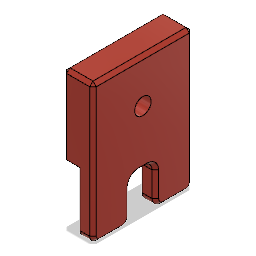
Bearing-mounting-blockV2 v6 (Autodesk Fusion 360 design; units mm, degrees)
Autodesk Fusion 360 part; units mm, degrees
sketch "Sketch1" plane through (0, 0, 0) normal (1, 0, 0) x (0, 0, -1)
  circle A0 centre (0, 0) radius 5
  line L0 (-30.15, -21.15) -> (30.15, -21.15)
  line L1 (30.15, -21.15) -> (30.15, 21.15)
  line L2 (-30.15, -21.15) -> (-30.15, 26.15)
  line L3 (-30.15, 26.15) -> (30.15, 26.15)
  line L4 (30.15, 26.15) -> (30.15, 21.15)
  dimension "d11" = 10
  dimension "d127" = 60.3
  dimension "d142" = 21.15
  dimension "d143" = 30.15
  measures "d11" diameter of A0
  measures "d127" distance of L2 L4
extrude "Extrude1" add sketch "Sketch1" along normal blind 8
sketch "Sketch16" plane through (0, -21.15, 0) normal (0, -1, 0) x (1, 0, 0)
  line L0 (0, 30.15) -> (0, -30.15)
  line L1 (0, -30.15) -> (8, -30.15)
  line L2 (8, -30.15) -> (8, 30.15)
  line L3 (8, 30.15) -> (0, 30.15)
  line L4 (4, 26.25) -> (4, -26.25) construction
  circle A0 centre (4, 26.25) radius 2.6
  circle A1 centre (4, -26.25) radius 2.6
  dimension "d144" = 4
  dimension "d145" = 52.5
  dimension "d146" = 5.2
  dimension "d147" = 5.2
  dimension "d148" = 26.25
  measures "d144" distance of origin L4
  measures "d146" diameter of A0
  measures "d147" diameter of A1
  measures "d148" distance of origin
extrude "Extrude17" cut sketch "Sketch16" against normal blind 7 contours A0 | A1
sketch "Sketch17" plane through (0, -14.15, 0) normal (0, -1, 0) x (1, 0, 0)
  circle A0 centre (4, 26.25) radius 2.6
  line L0 (4, 26.25) -> (4, -26.25)
  circle A1 centre (4, 26.25) radius 2
  circle A2 centre (4, -26.25) radius 2
  dimension "d151" = 52.5
  dimension "d152" = 4
  dimension "d153" = 4
  measures "d152" diameter of A2
  measures "d153" diameter of A1
extrude "Extrude18" cut sketch "Sketch17" against normal blind 10 contours A1 | A2
extrude "Extrude19" add 1 faces at (8, 1.9151, -21.7481) along direction (1, 0, 0) blind 10
sketch "Sketch18" plane through (0, -21.15, 0) normal (0, -1, 0) x (1, 0, 0)
  circle A0 centre (4, 26.25) radius 2.6
  circle A1 centre (4, -26.25) radius 2.6
  line L0 (0, 30.15) -> (0, -30.15)
  line L1 (0, -30.15) -> (18, -30.15)
  line L2 (18, -30.15) -> (18, 30.15)
  line L3 (18, 30.15) -> (0, 30.15)
  line L4 (18, 30.15) -> (8, 30.15)
  line L5 (8, 30.15) -> (8, -30.15)
  line L6 (8, -30.15) -> (18, -30.15)
  line L7 (18, -30.15) -> (18, 30.15)
  dimension "d159" = 10
  measures "d159" distance of L5 L7
extrude "Extrude20" add sketch "Sketch18" along normal blind 37 contours L1 L2 L3 L4 L5 L6 L7
sketch "Sketch19" plane through (18, 0, 0) normal (1, 0, 0) x (0, 0, -1)
  circle A0 centre (0, 0) radius 5
  line L0 (30.15, -58.15) -> (30.15, 26.15)
  line L1 (30.15, 26.15) -> (-30.15, 26.15)
  line L2 (-30.15, 26.15) -> (-30.15, -58.15)
  line L3 (-7.5, -58.15) -> (7.5, -58.15)
  line L4 (7.5, -53.15) -> (7.5, -38.15)
  line L5 (2.5, -33.15) -> (-2.5, -33.15)
  line L6 (-7.5, -38.15) -> (-7.5, -53.15)
  line L7 (12.5, -58.15) -> (26.15, -58.15)
  line L8 (30.15, -54.15) -> (30.15, 26.15)
  line L9 (30.15, 26.15) -> (-30.15, 26.15)
  line L10 (-30.15, 26.15) -> (-30.15, -54.15)
  arc A1 (-2.5, -33.15) -> (-7.5, -38.15) centre (-2.5, -38.15) ccw
  arc A2 (7.5, -38.15) -> (2.5, -33.15) centre (2.5, -38.15) ccw
  arc A3 (7.5, -53.15) -> (12.5, -58.15) centre (12.5, -53.15) ccw
  line L11 (-26.15, -58.15) -> (-12.5, -58.15)
  arc A4 (-12.5, -58.15) -> (-7.5, -53.15) centre (-12.5, -53.15) ccw
  line L12 (30.15, -58.15) -> (-30.15, -58.15)
  arc A5 (-30.15, -54.15) -> (-26.15, -58.15) centre (-26.15, -54.15) ccw
  arc A6 (26.15, -58.15) -> (30.15, -54.15) centre (26.15, -54.15) ccw
  dimension "d162" = 15
  dimension "d163" = 25
  dimension "d164" = 7.5
  dimension "d165" = 5
  dimension "d166" = 5
  dimension "d167" = 4
  dimension "d168" = 4
  measures "d164" distance of A0.centre
  measures "d165" radius of A1
  measures "d166" radius of A4
  measures "d167" radius of A5
  measures "d168" radius of A6
extrude "Extrude21" cut sketch "Sketch19" against normal up to surface (10 mm away) contours L0 L12 A6 | L3 L4 L5 L6 A1 A2 A3 A4 L12 | L2 L12 A5
chamfer "Chamfer1" distance 2 angle 45 32 edges at (18, 26.15, 0) (9, 26.15, 30.15) (0, 26.15, 0) (0, 2.5, 30.15) (18, -14, 30.15) (18, -56.9784, 28.9784) (18, -58.15, 19.325) (18, -56.6855, 8.9645) (18, -45.65, 7.5) (18, -34.6145, 6.0355) (18, -33.15, 0) (18, -34.6145, -6.0355) (18, -45.65, -7.5) (18, -56.6855, -8.9645) (18, -58.15, -19.325) (18, -56.9784, -28.9784) (18, -14, -30.15) (8, -37.65, 30.15) (8, -56.9784, 28.9784) (8, -58.15, 19.325) (8, -56.6855, 8.9645) (8, -45.65, 7.5) (8, -34.6145, 6.0355) (8, -33.15, 0) (8, -34.6145, -6.0355) (8, -45.65, -7.5) (8, -56.6855, -8.9645) (8, -58.15, -19.325) (8, -56.9784, -28.9784) (8, -37.65, -30.15) (0, 2.5, -30.15) (9, 26.15, -30.15)
equation "d143 = ( 60.3 / 2 ) * 1 mm"
equation "d148 = ( 52.5 / 2 ) * 1 mm"
